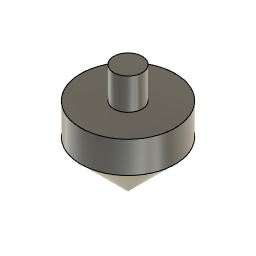
feet v2 (Autodesk Fusion 360 design; units mm, degrees)
Autodesk Fusion 360 part; units mm, degrees
sketch "Sketch1" plane through (0, 0, 0) normal (0, 0, 1) x (1, 0, 0)
  circle A0 centre (0, 0) radius 15
  dimension "d1" = 30
  constraint coincident A0.centre origin
  measures "d1" diameter of A0
extrude "Extrude1" add sketch "Sketch1" along normal blind 30
chamfer "Chamfer1" distance 15 angle 45 1 edges at (-13.9849, -5.4242, 0)
extrude "Extrude2" cut 1 faces at (3.8315, 5.6199, 30) along direction (0, 0, -1) blind 5
sketch "Sketch2" plane through (0, 0, 25) normal (0, 0, 1) x (-1, 0, 0)
  circle A0 centre (0, 0) radius 15
  circle A1 centre (0, 0) radius 4.518
  dimension "d7" = 9.036
  constraint coincident A0.centre A1.centre
  measures "d7" diameter of A1
extrude "Extrude3" add sketch "Sketch2" along normal blind 20 contours A1
extrude "Extrude4" cut 1 faces at (1.3657, -1.8727, 45) along direction (0, 0, -1) blind 10
equation "d7 = ( 4.518 * 2 ) * 1 mm"
